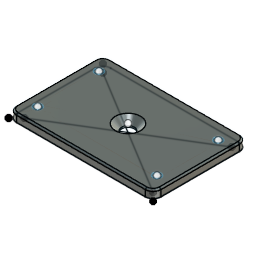
WeatherLox-Rain-Adapter (Autodesk Fusion 360 design; units mm, degrees)
Autodesk Fusion 360 part; units mm, degrees
note: some values were not read from the file. Set by a fixed rule: which sketch regions a step uses.
sketch "Skizze1" plane through (0, 0, 0) normal (0, 0, 1) x (1, 0, 0)
  line L0 (5, 0) -> (87, 0)
  line L1 (92, 5) -> (92, 55)
  line L2 (87, 60) -> (5, 60)
  line L3 (0, 55) -> (0, 5)
  arc A0 (92, 55) -> (87, 60) centre (87, 55) ccw
  arc A1 (87, 0) -> (92, 5) centre (87, 5) ccw
  arc A2 (5, 60) -> (0, 55) centre (5, 55) ccw
  arc A3 (0, 5) -> (5, 0) centre (5, 5) ccw
  line L4 (5, 55) -> (87, 5)
  line L5 (87, 55) -> (5, 5)
  point P0 (92, 0)
  point P1 (0, 60)
  dimension "d18" = 92
  dimension "d19" = 60
  dimension "d20" = 5
  dimension "d21" = 5
  dimension "d22" = 5
  dimension "d23" = 5
  constraint horizontal L0
  constraint vertical L1
  constraint horizontal L2
  constraint vertical L3
  constraint tangent L2 A0
  constraint tangent L1 A0
  constraint coincident P0 L1
  constraint coincident P0 L0
  constraint tangent L1 A1
  constraint tangent L0 A1
  constraint coincident P1 L2
  constraint coincident P1 L3
  constraint tangent L2 A2
  constraint tangent L3 A2
  constraint coincident origin L0
  constraint coincident origin L3
  constraint tangent L0 A3
  constraint tangent L3 A3
  constraint coincident A2.centre L4.start
  constraint coincident A1.centre L4.end
  constraint coincident A0.centre L5.start
  constraint coincident A3.centre L5.end
  measures "d18" distance of origin P0
  measures "d19" distance of origin P1
  measures "d20" radius of A0
  measures "d21" radius of A1
  measures "d22" radius of A2
  measures "d23" radius of A3
extrude "Extrusion2" add sketch "Skizze1" along normal blind 5
sketch "Skizze3" plane through (0, 0, 5) normal (0, 0, 1) x (-1, 0, 0)
  arc A0 (0, -5) -> (-5, 0) centre (-5, -5) ccw
  line L0 (-5, 0) -> (-87, 0)
  arc A1 (-87, 0) -> (-92, -5) centre (-87, -5) ccw
  line L1 (-92, -5) -> (-92, -55)
  arc A2 (-92, -55) -> (-87, -60) centre (-87, -55) ccw
  line L2 (-87, -60) -> (-5, -60)
  arc A3 (-5, -60) -> (0, -55) centre (-5, -55) ccw
  line L3 (0, -55) -> (0, -5)
  circle A4 centre (-8, -49.5) radius 2.25
  circle A5 centre (-8, -10.5) radius 2.25
  circle A6 centre (-84, -49.5) radius 2.25
  circle A7 centre (-84, -10.5) radius 2.25
  point P0 (-46, -30)
  dimension "d36" = 4.5
  dimension "d37" = 4.5
  dimension "d42" = 4.5
  dimension "d43" = 4.5
  measures "d36" diameter of A4
  measures "d37" diameter of A5
  measures "d42" diameter of A6
  measures "d43" diameter of A7
hole "Bohrung2" at (46, 30, 5) direction (0, 0, -1) diameter 8 depth 5 tip angle 118 countersink diameter 16 countersink angle 90
extrude "Extrusion3" cut sketch "Skizze3" against normal blind 10 contours A7
extrude "Extrusion4" cut sketch "Skizze3" against normal blind 10 contours A6
extrude "Extrusion5" cut sketch "Skizze3" against normal blind 10 contours A4
extrude "Extrusion6" cut sketch "Skizze3" against normal blind 10 contours A5
chamfer "Fase2" distance 1 angle 45 8 edges at (46, 0, 5) (90.5355, 1.4645, 5) (92, 30, 5) (90.5355, 58.5355, 5) (46, 60, 5) (1.4645, 58.5355, 5) (0, 30, 5) (1.4645, 1.4645, 5)
